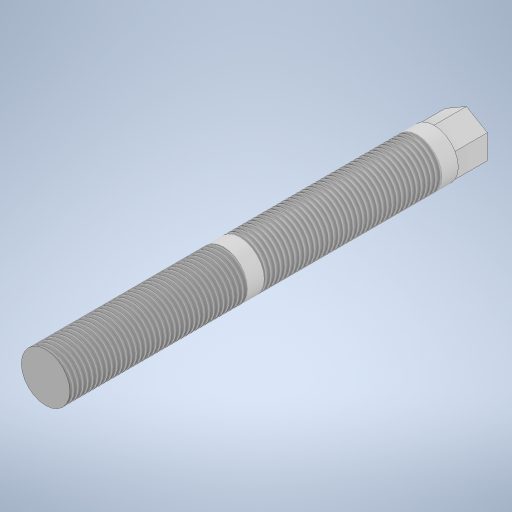
# Autodesk Inventor part: śruba
Saved by Autodesk Inventor 2024 (Build 280153000, 153)
## iProperties
Created: 2024-09-18
Part Number: śruba
Material: Ogólny
Document SubType Name: Modeling
Designer: JEDEN
Density: 1 g/cm^3
Appearance: Domyślna
Author: JEDEN
Autodesk Inventor part; units mm, degrees
ref_plane "YZ Plane" through (0, 0, 0) normal (1, 0, 0) x (0, 1, 0)
ref_plane "XZ Plane" through (0, 0, 0) normal (0, 1, 0) x (-1, 0, 0)
ref_plane "XY Plane" through (0, 0, 0) normal (0, 0, 1) x (1, 0, 0)
sketch "Szkic1" plane through (0, 0, 0) normal (0, 0, 1) x (1, 0, 0)
  circle A0 centre (-4.3569, 3.3954) radius 15
  point P0 (0, 0)
  dimension "d0" = 30
  constraints: 1 centre point
  measures "d0" diameter of A0
extrude "Wyciągnięcie proste1" add sketch "Szkic1" along normal blind 240
thread "Gwint1" size "TR30x3" class "7e" standard "ISO Metric Trapezoidal Threads" length 230 offset 130
thread "Gwint2" size "TR30x3" class "7e" standard "ISO Metric Trapezoidal Threads" length 110 offset 10
sketch "Szkic2" plane through (-4.3569, 3.3954, 0) normal (0, 0, -1) x (-1, 0, 0)
  circle A0 centre (0, 0) radius 15 projected
  line L0 (0, 15) -> (12.9904, 7.5)
  line L1 (12.9904, 7.5) -> (12.9904, -7.5)
  line L2 (12.9904, -7.5) -> (0, -15)
  line L3 (0, -15) -> (-12.9904, -7.5)
  line L4 (-12.9904, -7.5) -> (-12.9904, 7.5)
  line L5 (-12.9904, 7.5) -> (0, 15)
  point P0 (-4.3569, -3.3954)
  dimension "d9" = 360
  constraints: 12 end point, 3 parallel, 1 coincident, 1 vertical, 1 vertical alignment, 8 other
extrude "Wyciągnięcie proste2" add sketch "Szkic2" along normal blind 20 contours L1 L2 L3 L4 L5 L0
